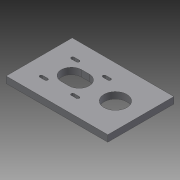
# Autodesk Inventor part: WoodD_Extruder_Side_Motor
Saved by Autodesk Inventor 2014 SP2 (Build 180246200, 246)
## iProperties
Created: 2014-09-30
Part Number: WoodD_Extruder_Side_Motor
Material: Generic
Document SubType Name: Modeling
Designer: ThatOtherGuy
Density: 1 g/cm^3
Appearance: Default
Author: ThatOtherGuy
Autodesk Inventor part; units mm, degrees
ref_plane "YZ Plane" through (0, 0, 0) normal (1, 0, 0) x (0, 1, 0)
ref_plane "XZ Plane" through (0, 0, 0) normal (0, 1, 0) x (-1, 0, 0)
ref_plane "XY Plane" through (0, 0, 0) normal (0, 0, 1) x (1, 0, 0)
sketch "Sketch1" plane through (0, 0, 0) normal (0, 0, 1) x (1, 0, 0)
  line L0 (0, 0) -> (100, 0)
  line L1 (100, 0) -> (100, 65)
  line L2 (100, 65) -> (0, 65)
  line L3 (0, 65) -> (0, 0)
  line L4 (17.5, 48) -> (22.5, 48) construction
  line L5 (17.5, 46.5) -> (22.5, 46.5)
  line L6 (22.5, 49.5) -> (17.5, 49.5)
  arc A0 (17.5, 49.5) -> (17.5, 46.5) centre (17.5, 48) ccw
  arc A1 (22.5, 46.5) -> (22.5, 49.5) centre (22.5, 48) ccw
  line L7 (53.5, 48) -> (48.5, 48) construction
  line L8 (53.5, 49.5) -> (48.5, 49.5)
  line L9 (48.5, 46.5) -> (53.5, 46.5)
  arc A2 (53.5, 46.5) -> (53.5, 49.5) centre (53.5, 48) ccw
  arc A3 (48.5, 49.5) -> (48.5, 46.5) centre (48.5, 48) ccw
  line L10 (17.5, 17) -> (22.5, 17) construction
  line L11 (17.5, 15.5) -> (22.5, 15.5)
  line L12 (22.5, 18.5) -> (17.5, 18.5)
  arc A4 (17.5, 18.5) -> (17.5, 15.5) centre (17.5, 17) ccw
  arc A5 (22.5, 15.5) -> (22.5, 18.5) centre (22.5, 17) ccw
  line L13 (48.5, 17) -> (53.5, 17) construction
  line L14 (48.5, 15.5) -> (53.5, 15.5)
  line L15 (53.5, 18.5) -> (48.5, 18.5)
  arc A6 (48.5, 18.5) -> (48.5, 15.5) centre (48.5, 17) ccw
  arc A7 (53.5, 15.5) -> (53.5, 18.5) centre (53.5, 17) ccw
  line L16 (31.75, 32.5) -> (39.25, 32.5) construction
  line L17 (31.75, 22.5) -> (39.25, 22.5)
  line L18 (39.25, 42.5) -> (31.75, 42.5)
  arc A8 (31.75, 42.5) -> (31.75, 22.5) centre (31.75, 32.5) ccw
  arc A9 (39.25, 22.5) -> (39.25, 42.5) centre (39.25, 32.5) ccw
  circle A10 centre (75, 32.5) radius 11.25
  point P0 (20, 48)
  point P1 (51, 48)
  point P2 (20, 17)
  point P3 (51, 17)
  point P4 (35.5, 32.5)
  point P5 (0, 32.5)
  dimension "d0" = 65
  dimension "d1" = 100
  dimension "d2" = 1.5
  dimension "d3" = 5
  dimension "d4" = 31
  dimension "d5" = 31
  dimension "d6" = 20
  dimension "d7" = 15.5
  dimension "d8" = 15.5
  dimension "d9" = 7.5
  dimension "d10" = 20
  dimension "d11" = 75
  dimension "d12" = 22.5
  constraints: 48 end point, 20 point on circle, 20 tangent, 12 parallel, 11 centre point, 6 midpoint, 4 horizontal alignment, 3 equal length, 3 equal radius, 2 vertical alignment, 1 horizontal, 1 perpendicular
  measures "d0" distance of L2.end L0.start
  measures "d1" distance of L0.start L0.end
  measures "d2" radius of A1
  measures "d3" distance of L4.start L4.end
  measures "d4" distance of point (20, 17) point (20, 48)
  measures "d5" distance of point (20, 48) point (51, 48)
  measures "d6" distance between parallel lines of L17 L18
  measures "d7" horizontal distance of point (20, 48) point (35.5, 32.5)
  measures "d8" horizontal distance of point (35.5, 32.5) point (20, 48)
  measures "d9" distance of L16.start L16.end
  measures "d10" distance from line of L3 point (20, 17)
  measures "d11" distance from line of L3 A10.centre
  measures "d12" diameter of A10
extrude "Extrusion1" add sketch "Sketch1" along normal blind 6.35
equation "\"d5\" = d4"
equation "\"d7\" = 0.5 * d4"
equation "\"d8\" = 0.5 * d5"
equation "\"d13\" = THICKB"
equation "\"THICKA\" = 3.175"
equation "\"THICKB\" = 6.35"
equation "\"THICKC\" = 12.7"
body "Solid1"
